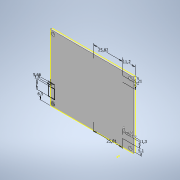
# Autodesk Inventor part: lunchpad
Saved by Autodesk Inventor 2022 (Build 260153000, 153)
## iProperties
Created: 2021-08-24
Part Number: lunchpad
Material: Generic
Document SubType Name: Modeling
Designer: jonar
Density: 1 g/cm^3
Appearance: Default
Author: jonar
Autodesk Inventor part; units mm, degrees
ref_plane "YZ Plane" through (0, 0, 0) normal (1, 0, 0) x (0, 1, 0)
ref_plane "XZ Plane" through (0, 0, 0) normal (0, 1, 0) x (-1, 0, 0)
ref_plane "XY Plane" through (0, 0, 0) normal (0, 0, 1) x (1, 0, 0)
sketch "card" plane through (0, 0, 0) normal (0, 0, 1) x (1, 0, 0)
  line L0 (-59.3579, 68.5808) -> (-59.3579, 10.0008)
  line L1 (-59.3579, 10.0008) -> (14.2921, 10.0008)
  line L2 (14.2921, 10.0008) -> (14.2921, 68.5808)
  line L3 (14.2921, 68.5808) -> (-59.3579, 68.5808)
  circle A0 centre (11.6671, 65.9558) radius 1.575
  circle A1 centre (11.6671, 12.6258) radius 1.575
  circle A2 centre (-56.7329, 65.9558) radius 1.575
  circle A3 centre (-56.7329, 12.6258) radius 1.575
  point P0 (0, 0)
  dimension "d1" = 58.58
  dimension "d2" = 73.65
  dimension "d4" = 2.625
  dimension "d5" = 3.15
  constraints: 8 end point, 4 centre point, 2 perpendicular, 1 vertical
  measures "d1" distance of L1.end L2.end
  measures "d2" distance of L2.end L0.start
  measures "d4" distance from line of L2 A0.centre
  measures "d5" diameter of A0
extrude "main_board" add sketch "card" along normal blind 1.6
sketch "front_components" plane through (0, 0, 1.6) normal (0, 0, 1) x (1, 0, 0)
  line L0 (-55.4979, 24.5008) -> (-61.1579, 24.5008)
  line L1 (-61.1579, 24.5008) -> (-61.1579, 16.5008)
  line L2 (-61.1579, 16.5008) -> (-55.4979, 16.5008)
  line L3 (-55.4979, 16.5008) -> (-55.4979, 24.5008)
  line L4 (-59.3579, 10.0008) -> (14.2921, 10.0008) projected
  line L5 (-59.3579, 68.5808) -> (-59.3579, 10.0008) projected
  point P0 (0, 0)
  dimension "d19" = 6.5
  dimension "d20" = 8
  dimension "d21" = 1.8
  dimension "d22" = 5.66
  constraints: 8 end point, 2 perpendicular, 1 horizontal, 1 vertical
  measures "d19" distance between parallel lines of L2 L4
  measures "d20" distance between parallel lines of L0 L2
  measures "d21" distance between parallel lines of L5 L1
  measures "d22" distance between parallel lines of L3 L1
sketch "back_components" plane through (0, 0, 0) normal (0, 0, -1) x (-1, 0, 0)
  line L0 (-3.0921, 63.3708) -> (22.7279, 63.3708)
  line L1 (22.7279, 63.3708) -> (22.7279, 58.3708)
  line L2 (22.7279, 58.3708) -> (-3.0921, 58.3708)
  line L3 (-3.0921, 58.3708) -> (-3.0921, 63.3708)
  line L4 (-2.9921, 20.1008) -> (22.8179, 20.1008)
  line L5 (22.8179, 20.1008) -> (22.8179, 15.1008)
  line L6 (22.8179, 15.1008) -> (-2.9921, 15.1008)
  line L7 (-2.9921, 15.1008) -> (-2.9921, 20.1008)
  line L8 (-14.2921, 68.5808) -> (59.3579, 68.5808) projected
  line L9 (-14.2921, 10.0008) -> (-14.2921, 68.5808) projected
  line L10 (59.3579, 10.0008) -> (-14.2921, 10.0008) projected
  point P0 (0, 0)
  dimension "d23" = 5.21
  dimension "d24" = 11.2
  dimension "d25" = 5.1
  dimension "d26" = 11.3
  dimension "d27" = 5
  dimension "d28" = 5
  dimension "d29" = 25.82
  dimension "d30" = 25.81
  constraints: 16 end point, 3 parallel, 2 horizontal, 2 perpendicular
  measures "d23" distance between parallel lines of L8 L0
  measures "d24" distance between parallel lines of L9 L3
  measures "d25" distance between parallel lines of L10 L6
  measures "d26" distance between parallel lines of L9 L7
  measures "d27" distance between parallel lines of L6 L4
  measures "d28" distance between parallel lines of L0 L2
  measures "d29" distance between parallel lines of L1 L3
  measures "d30" distance between parallel lines of L5 L7
body "Solid1"
